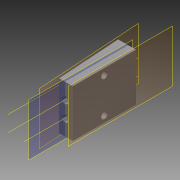
# Autodesk Inventor part: loop holder
Saved by Autodesk Inventor 2015 (Build 190159000, 159)
## iProperties
Created: 2014-05-22
Part Number: loop holder
Material: Generic
Document SubType Name: Modeling
Designer: jad211
Density: 1 g/cm^3
Appearance: Default
Author: jad211
Autodesk Inventor part; units mm, degrees
ref_plane "XZ Plane" through (0, 0, 0) normal (0, 1, 0) x (-1, 0, 0)
ref_plane "XY Plane" through (0, 0, 0) normal (0, 0, 1) x (1, 0, 0)
sketch "Sketch1" plane through (0, 0, 0) normal (0, 1, 0) x (-1, 0, 0)
  line L0 (-5, 7.5) -> (5, 7.5)
  line L1 (5, 7.5) -> (5, -7.5)
  line L2 (5, -7.5) -> (-5, -7.5)
  line L3 (-5, -7.5) -> (-5, 7.5)
  line L4 (-5, 7.5) -> (5, -7.5) construction
  line L5 (5, 7.5) -> (-5, -7.5) construction
  line L6 (-2.5, 2.5) -> (2.5, 2.5) construction
  line L7 (2.5, 2.5) -> (2.5, -2.5) construction
  line L8 (2.5, -2.5) -> (-2.5, -2.5) construction
  line L9 (-2.5, -2.5) -> (-2.5, 2.5) construction
  line L10 (-2.5, 2.5) -> (2.5, -2.5) construction
  line L11 (2.5, 2.5) -> (-2.5, -2.5) construction
  circle A0 centre (2.5, -2.5) radius 1.1
  circle A1 centre (2.5, 2.5) radius 1.1
  circle A2 centre (-2.5, -2.5) radius 1.1
  circle A3 centre (-2.5, 2.5) radius 1.1
  point P0 (0, 0)
  dimension "d6" = 2.2
  dimension "d7" = 2.2
  dimension "d8" = 2.2
  dimension "d9" = 2.2
  dimension "d10" = 10
  dimension "d11" = 15
  dimension "d12" = 5
  dimension "d13" = 5
  constraints: 24 end point, 4 centre point, 4 coincident, 4 midpoint, 4 parallel, 3 perpendicular, 1 horizontal
  measures "d6" diameter of A0
  measures "d7" diameter of A1
  measures "d8" diameter of A3
  measures "d9" diameter of A2
  measures "d10" distance of L1.end L2.end
  measures "d11" distance of L0.end L1.end
  measures "d12" distance of L6.start L6.end
  measures "d13" distance of L6.end L7.end
extrude "Extrusion3" add sketch "Sketch1" along normal mid plane 20
ref_plane "Work Plane2" through (2.5, 10, -2.5) normal (-1, 0, 0) x (0, -1, 0)
ref_plane "Work Plane4" through (0, 0, 0) normal (0.997813, 0.0660998, 0) x (0, 0, 1)
split "Split2" plane through (0, 0, 0) removes the side toward (-0.997813, -0.0660998, 0)
ref_plane "Work Plane5" through (5, -10, -7.5) normal (1, 0, 0) x (0, 0, -1)
sketch "Sketch3" plane through (5, -10, -7.5) normal (1, 0, 0) x (0, 0, -1)
  line L0 (-2, 10) -> (-13, 10) construction
  circle A0 centre (-13, 10) radius 1
  circle A1 centre (-2, 10) radius 1
  point P0 (-7.5, 10)
  dimension "d21" = 5.5
  dimension "d22" = 5.5
  dimension "d23" = 2
  dimension "d24" = 2
  constraints: 2 centre point, 2 coincident, 2 end point
  measures "d21" distance of L0.end point (-7.5, 10)
  measures "d22" distance of point (-7.5, 10) L0.start
  measures "d23" diameter of A0
  measures "d24" diameter of A1
extrude "Extrusion4" cut sketch "Sketch3" against normal through all
split body "Split5" result two bodies by plane through (2.5, 10, -2.5) normal (-1, 0, 0) first body at (0.9582, -6.9004, 1.6335)
thread "Thread1" size "M2x0.4" class "6H" standard "ANSI Metric M Profile" full length
thread "Thread2" size "M2x0.4" class "6H" standard "ANSI Metric M Profile" full length
equation "\"d7\" = d6"
equation "\"d8\" = d7"
equation "\"d9\" = d6"
equation "\"d22\" = d21"
equation "\"d24\" = d23"
body "Solid11"
body "Solid12"
